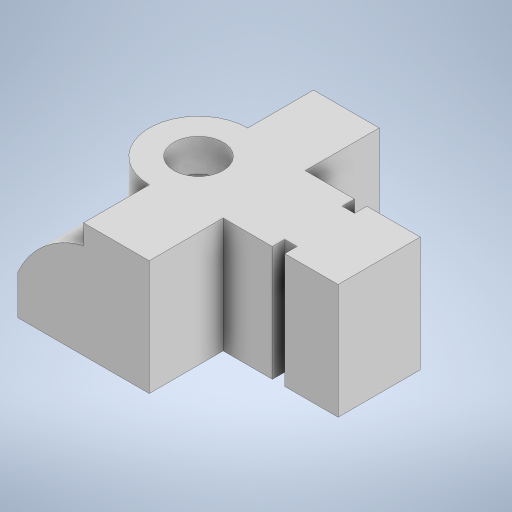
# Autodesk Inventor part: Pieza6-Tarea1
Saved by Autodesk Inventor 2024 (Build 280153000, 153)
## iProperties
Created: 2024-02-16
Part Number: Pieza6-Tarea1
Material: Genérico
Document SubType Name: Modeling
Designer: Diegolap
Density: 1 g/cm^3
Appearance: Valor por defecto
Mass: 230.372 g
Surface Area: 283.237 cm^2
Volume: 230.372 cm^3
Author: Diegolap
Autodesk Inventor part; units mm, degrees
ref_plane "YZ Plane" through (0, 0, 0) normal (1, 0, 0) x (0, 1, 0)
ref_plane "XZ Plane" through (0, 0, 0) normal (0, 1, 0) x (-1, 0, 0)
ref_plane "XY Plane" through (0, 0, 0) normal (0, 0, 1) x (1, 0, 0)
sketch "Boceto1" plane through (0, 0, 0) normal (0, 1, 0) x (-1, 0, 0)
  line L0 (25.4, 44.45) -> (-25.4, 44.45)
  line L1 (-25.4, 44.45) -> (-25.4, -44.45)
  line L2 (-25.4, -44.45) -> (25.4, -44.45)
  line L3 (25.4, -44.45) -> (25.4, 44.45)
  line L4 (25.4, 44.45) -> (-25.4, -44.45) construction
  line L5 (-25.4, 44.45) -> (25.4, -44.45) construction
  line L6 (-25.4, -15.875) -> (-69.85, -15.875)
  line L7 (-69.85, -15.875) -> (-69.85, 15.875)
  line L8 (-69.85, 15.875) -> (-25.4, 15.875)
  line L9 (-25.4, 15.875) -> (-25.4, -15.875)
  line L10 (-25.4, 44.45) -> (0, 44.45)
  line L11 (0, 44.45) -> (0, -44.45)
  line L12 (0, -44.45) -> (-25.4, -44.45)
  line L13 (-25.4, -44.45) -> (-25.4, 44.45)
  line L14 (-25.4, 15.875) -> (-43.4008, 15.875)
  line L15 (-25.4, 15.875) -> (-44.45, 15.875)
  line L16 (-44.45, 15.875) -> (-49.2125, 15.875)
  line L17 (-49.2125, 15.875) -> (-44.45, 15.875)
  line L18 (-44.45, 15.875) -> (-44.45, 11.1125)
  line L19 (-44.45, 11.1125) -> (-49.2125, 11.1125)
  line L20 (-49.2125, 11.1125) -> (-49.2125, 15.875)
  line L21 (-49.2125, -15.875) -> (-44.45, -15.875)
  line L22 (-44.45, -15.875) -> (-44.45, -11.1125)
  line L23 (-44.45, -11.1125) -> (-49.2125, -11.1125)
  line L24 (-49.2125, -11.1125) -> (-49.2125, -15.875)
  point P0 (0, 0)
  dimension "d0" = 28.575
  dimension "d1" = 28.575
  dimension "d2" = 31.75
  dimension "d3" = 50.8
  dimension "d4" = 44.45
  dimension "d5" = 19.05
  dimension "d6" = 4.7625
  dimension "d7" = 4.7625
  dimension "d8" = 4.7625
  dimension "d9" = 4.7625
  dimension "d10" = 19.05
  constraints: 50 end point, 10 parallel, 5 horizontal, 5 perpendicular, 5 point on line, 3 midpoint
  measures "d0" distance of L0.end L8.end
  measures "d1" distance of L1.end L6.start
  measures "d2" distance of L8.end L6.start
  measures "d3" distance of L0.start L0.end
  measures "d4" distance of L7.end L8.end
  measures "d5" distance of L8.end L15.end
  measures "d6" distance of L15.end L16.end
  measures "d7" distance of L19.end L16.end
  measures "d8" distance of L22.end L23.end
  measures "d9" distance of L23.end L21.start
  measures "d10" distance between parallel lines of L13 L22
extrude "Extrusión1" add sketch "Boceto1" along normal blind 44.45 contours L11 L2 L1 L0 | L1 L6 L22 L23 L24 L7 L8 L20 L19 L18
sketch "Boceto2" plane through (0, 0, 44.45) normal (0, 0, 1) x (1, 0, 0)
  line L0 (0, 0) -> (25.4, 0) projected
  line L1 (25.4, 0) -> (9.525, 0)
  circle A0 centre (9.525, 0) radius 38.1
  line L2 (25.4, 0) -> (-25.4, 0)
  line L3 (-25.4, 0) -> (-25.4, 15.2268)
  line L4 (0, 0) -> (0, 36.8902)
  dimension "d13" = 15.875
  dimension "d14" = 76.2
  dimension "d15" = 50.8
  constraints: 8 end point, 2 point on circle, 2 point on line, 1 centre point, 1 coincident, 1 perpendicular, 1 vertical
  measures "d13" distance of L1.end L0.end
  measures "d14" diameter of A0
  measures "d15" distance of L0.end L2.end
extrude "Extrusión2" add sketch "Boceto2" against normal blind 88.9 contours L4 L2 L3 A0 picked at (-16.9333, 5.0756)
sketch "Boceto3" plane through (0, 44.45, 0) normal (0, 1, 0) x (1, 0, 0)
  circle A0 centre (0, 0) radius 19.05
  circle A1 centre (0, 0) radius 9.525
  dimension "d18" = 38.1
  dimension "d19" = 19.05
  constraints: 2 centre point, 2 coincident
  measures "d18" diameter of A0
  measures "d19" diameter of A1
extrude "Extrusión3" add sketch "Boceto3" against normal blind 25.4
sketch "Boceto4" plane through (0, 44.45, 0) normal (0, 1, 0) x (1, 0, 0)
  circle A0 centre (0, 0) radius 9.525
  dimension "d22" = 19.05
  constraints: 1 centre point, 1 coincident
  measures "d22" diameter of A0
extrude "Extrusión4" cut sketch "Boceto4" against normal blind 12.7
